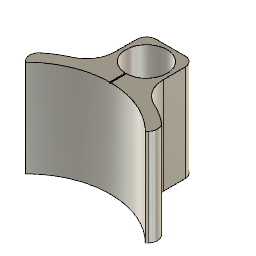
AvionicsTubeAttachment (Autodesk Fusion 360 design; units mm, degrees)
Autodesk Fusion 360 part; units mm, degrees
sketch "Sketch1" plane through (0, 0, 0) normal (0, 0, 1) x (1, 0, 0)
  circle A0 centre (0, 0) radius 44.45
  arc A1 (35.921, 35.921) -> (-35.921, 35.921) centre (0, 0) ccw
  line L0 (0, 0) -> (35.921, 35.921) construction
  line L1 (0, 0) -> (-35.921, 35.921) construction
  line L2 (-35.921, 35.921) -> (-31.4309, 31.4309) construction
  line L3 (-35.921, 35.921) -> (-31.4309, 31.4309)
  line L4 (31.4309, 31.4309) -> (35.921, 35.921)
  line L5 (0, 0) -> (0, 50.8) construction
  line L6 (0, 50.8) -> (-31.4309, 31.4309) construction
  line L7 (0, 50.8) -> (31.4309, 31.4309) construction
  line L8 (-12.7, 76.2) -> (12.7, 76.2)
  line L9 (12.7, 76.2) -> (12.7, 50.8)
  line L10 (12.7, 50.8) -> (-12.7, 50.8) construction
  line L11 (-12.7, 50.8) -> (-12.7, 76.2)
  line L12 (-12.7, 50.8) -> (-12.7, 49.1869)
  line L13 (12.7, 50.8) -> (12.7, 49.1869)
  line L14 (-12.7, 63.5) -> (12.7, 63.5) construction
  circle A2 centre (0, 63.5) radius 10.795
  point P0 (-31.4309, 31.4309)
  point P1 (-12.7, 49.1869)
  point P2 (12.7, 49.1869)
  point P3 (-12.7, 63.5)
  point P4 (12.7, 63.5)
  dimension "d1" = 88.9
  dimension "d2" = 90
  dimension "d3" = 6.35
  dimension "d6" = 25.4
  dimension "d7" = 25.4
  dimension "d8" = 21.59
  constraint coincident A0.centre A1.centre
  constraint coincident A0 P0
  constraint coincident L1 P0
  constraint coincident P0 L2.end
  constraint coincident A0 L4.start
  constraint coincident L0 L4.start
  constraint vertical L5
  constraint equal L6 L7
  constraint midpoint A1 L5.end
  constraint horizontal L8
  constraint vertical L9
  constraint horizontal L10
  constraint vertical L11
  constraint midpoint L5.end L10
  constraint coincident A1 P1
  constraint perpendicular L10 L12
  constraint coincident A1 P2
  constraint perpendicular L10 L13
  constraint coincident P1 L12.end
  constraint coincident P2 L13.end
  constraint coincident L11 P3
  constraint midpoint L11 P3
  constraint midpoint L9 P4
  constraint coincident P3 L14.start
  constraint coincident P4 L14.end
  constraint midpoint L14 A2.centre
  measures "d1" diameter of A0
  measures "d2" angle of L0 L1
  measures "d3" distance of A1.end P0
  measures "d6" distance of L8.start L8.end
  measures "d7" distance of L8.end L9.end
  measures "d8" diameter of A2
extrude "Extrude2" add sketch "Sketch1" along normal blind 50.8 contours A0 A1 L3 L4 | A1 L8 L9 L11 L12 L13
fillet "Fillet1" radius 5 2 edges at (-35.921, 35.921, 25.4) (35.921, 35.921, 25.4)
fillet "Fillet2" radius 15 2 edges at (-12.7, 49.1869, 25.4) (12.7, 49.1869, 25.4)
fillet "Fillet3" radius 5 2 edges at (-12.7, 76.2, 25.4) (12.7, 76.2, 25.4)
sketch "Sketch4" plane through (0, 76.2, 0) normal (0, 1, 0) x (-1, 0, 0)
  line L0 (-7.7, 50.8) -> (-7.7, 0)
  line L1 (-7.7, 0) -> (7.7, 0)
  line L2 (7.7, 0) -> (7.7, 50.8)
  line L3 (7.7, 50.8) -> (-7.7, 50.8)
  line L4 (0, 0) -> (0, 16.9333) construction
  line L5 (0, 16.9333) -> (0, 33.8667) construction
  line L6 (0, 33.8667) -> (0, 50.8) construction
  circle A0 centre (0, 16.9333) radius 1.778
  circle A1 centre (0, 33.8667) radius 1.778
  dimension "d17" = 3.556
  dimension "d18" = 3.556
  constraint coincident L4.start origin
  constraint perpendicular L1 L4
  constraint parallel L4 L5
  constraint midpoint L3 L6.end
  constraint equal L5 L6
  constraint equal L4 L5
  constraint coincident L4.end L5.start
  constraint coincident L5.end L6.start
  measures "d17" diameter of A0
  measures "d18" diameter of A1
extrude "Extrude3" cut sketch "Sketch4" along normal up to surface contours A0 | A1 end surface at (10.7414, 62.4252, 33.8667)
sketch "Sketch6" plane through (0, 0, 50.8) normal (0, 0, 1) x (-1, 0, 0)
  arc A0 (-12.7, -71.2) -> (-7.7, -76.2) centre (-7.7, -71.2) ccw
  line L0 (-7.7, -76.2) -> (7.7, -76.2)
  arc A1 (7.7, -76.2) -> (12.7, -71.2) centre (7.7, -71.2) ccw
  line L1 (12.7, -71.2) -> (12.7, -59.6854)
  arc A2 (21.3854, -46.0793) -> (12.7, -59.6854) centre (27.7, -59.6854) ccw
  arc A3 (21.3854, -46.0793) -> (31.7848, -39.6278) centre (0, 0) ccw
  arc A4 (31.7848, -39.6278) -> (32.1919, -32.1919) centre (28.6564, -35.7275) ccw
  line L2 (32.1919, -32.1919) -> (31.4309, -31.4309)
  arc A5 (-31.4309, -31.4309) -> (31.4309, -31.4309) centre (0, 0) ccw
  line L3 (-31.4309, -31.4309) -> (-32.1919, -32.1919)
  arc A6 (-32.1919, -32.1919) -> (-31.7848, -39.6278) centre (-28.6564, -35.7275) ccw
  arc A7 (-31.7848, -39.6278) -> (-21.3854, -46.0793) centre (0, 0) ccw
  arc A8 (-12.7, -59.6854) -> (-21.3854, -46.0793) centre (-27.7, -59.6854) ccw
  line L4 (-12.7, -59.6854) -> (-12.7, -71.2)
  circle A9 centre (0, -63.5) radius 10.795
  line L5 (0, -52.705) -> (0, -44.45)
  circle A10 centre (0, -63.5) radius 10.795
  circle A11 centre (0, 0) radius 44.45
  line L6 (0.25, -52.705) -> (-0.25, -52.705)
  line L7 (-0.25, -52.705) -> (-0.25, -44.45)
  line L8 (-0.25, -44.45) -> (0.25, -44.45)
  line L9 (0.25, -44.45) -> (0.25, -52.705)
  line L10 (0, 0) -> (0, -50.8)
  dimension "d22" = 0.5
  constraint vertical L5
  constraint coincident L5.start A10
  constraint coincident L5.end A11
  constraint horizontal L6
  constraint vertical L7
  constraint horizontal L8
  constraint vertical L9
  constraint midpoint L5.start L6
  constraint midpoint L5.end L8
  constraint collinear L5 L10
  measures "d22" distance of L6.start L6.end
extrude "Extrude4" cut sketch "Sketch6" against normal blind 0.5 contours L5 L6 L8 L9 L10 | L5 L6 L7 L8 L10
